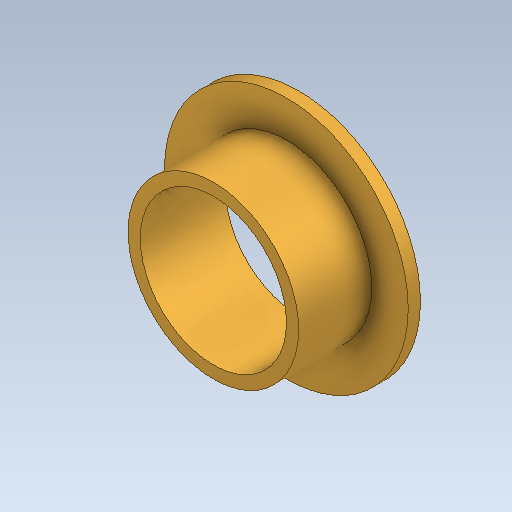
# Autodesk Inventor part: ドライメッシュw6f12-14a
Saved by Autodesk Inventor 2020.4 (Build 244396000, 396)
## iProperties
Created: 2020-04-12
Part Number: ドライメッシュw6f12-14a
Material: 真鍮、ソフト イエロー
Document SubType Name: Modeling
Designer: happy
Density: 8.47 g/cm^3
Appearance: 真鍮 - サテン
Mass: 3.77852 g
Surface Area: 9.92743 cm^2
Volume: 0.446106 cm^3
Author: happy
Autodesk Inventor part; units mm, degrees
ref_plane "YZ Plane" through (0, 0, 0) normal (1, 0, 0) x (0, 1, 0)
ref_plane "XZ Plane" through (0, 0, 0) normal (0, 1, 0) x (-1, 0, 0)
ref_plane "XY Plane" through (0, 0, 0) normal (0, 0, 1) x (1, 0, 0)
sketch "スケッチ1" plane through (0, 0, 0) normal (0, 0, 1) x (1, 0, 0)
  circle A0 centre (0, 0) radius 6
  circle A1 centre (0, 0) radius 7
  circle A2 centre (0, 0) radius 10
  dimension "d0" = 12
  dimension "d1" = 14
  dimension "d2" = 20
  constraints: 3 centre point, 3 coincident
  measures "d0" diameter of A0
  measures "d1" diameter of A1
  measures "d2" diameter of A2
extrude "押し出し1" add sketch "スケッチ1" along normal blind 1 contours A2
extrude "押し出し2" add sketch "スケッチ1" along normal blind 7 contours A1
